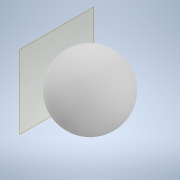
# Autodesk Inventor part: Ручка-09
Saved by Autodesk Inventor 2022 (Build 260153000, 153)
## iProperties
Created: 2021-12-02
Part Number: Ручка-09
Material: Типовые
Document SubType Name: Modeling
Designer: Украинцев
Density: 1 g/cm^3
Appearance: По умолчанию
Author: Украинцев
Autodesk Inventor part; units mm, degrees
ref_plane "XZ Plane" through (0, 0, 0) normal (0, 1, 0) x (-1, 0, 0)
ref_plane "XY Plane" through (0, 0, 0) normal (0, 0, 1) x (1, 0, 0)
sketch "Эскиз1" plane through (0, 0, 0) normal (0, 1, 0) x (-1, 0, 0)
  arc A0 (-15, 0) -> (15, 0) centre (0, 0) ccw
  line L0 (15, 0) -> (-15, 0)
  dimension "d0" = 30
  constraints: 2 end point, 2 point on circle, 1 centre point, 1 coincident, 1 horizontal
  measures "d0" diameter of A0
revolve "Вращение1" add sketch "Эскиз1" angle 360 about axis through (-15, 0, 0) along (1, 0, 0)
ref_plane "РабПлоскость1" through (-15, 0, 0) normal (1, 0, 0) x (0, 1, 0)
sketch "Эскиз2" plane through (-15, 0, 0) normal (1, 0, 0) x (0, 1, 0)
  point P0 (0, 0)
  point P1 (0, 0)
  constraints: 1 coincident
hole "Отверстие1" at (-15, 0, 0) direction (1, 0, 0) diameter 8.376 depth 22 tip angle 118 counterbore diameter 12 counterbore depth 4 thread size "M10x1.5" class "6H" standard "ISO Metric profile"
chamfer "Фаска1" distance 1.6 angle 45 1 edges at (-11, 0, -4.188)
